Autodesk Fusion 360 part; units mm, degrees
(part 2 of 2)
  spline S93 degree 3 poles (-0.4829, 17.1605) (-0.5355, 17.2267) (-0.6438, 17.3632) (-0.6565, 17.5373) (-0.663, 17.6271) knots 0 0 0 0 0.024747 0.051056 0.051056 0.051056 0.051056
  spline S94 degree 3 poles (-0.663, 17.6271) (-0.6569, 17.7139) (-0.645, 17.8842) (-0.5509, 18.0265) (-0.5048, 18.0964) knots 0 0 0 0 0.025614 0.050281 0.050281 0.050281 0.050281
  spline S95 degree 3 poles (-0.5048, 18.0964) (-0.4337, 18.1672) (-0.2885, 18.3119) (-0.0839, 18.33) (0.0205, 18.3392) knots 0 0 0 0 0.029141 0.059529 0.059529 0.059529 0.059529
  line L42 (4.4066, 19.7731) -> (4.2483, 19.7731)
  line L43 (4.2483, 19.7731) -> (4.2483, 21.7813)
  line L44 (4.2483, 21.7813) -> (4.4939, 21.7813)
  line L45 (4.4939, 21.7813) -> (4.4939, 20.2164)
  spline S96 degree 3 poles (4.4939, 20.2164) (4.5274, 20.2456) (4.5999, 20.3087) (4.6822, 20.3587) (4.7265, 20.3856) knots 0 0 0 0 0.013289 0.028808 0.028808 0.028808 0.028808
  spline S97 degree 3 poles (4.7265, 20.3856) (4.7715, 20.4114) (4.855, 20.4592) (4.944, 20.4957) (4.985, 20.5125) knots 0 0 0 0 0.015536 0.028826 0.028826 0.028826 0.028826
  line L46 (4.985, 20.5125) -> (4.985, 20.2751)
  spline S98 degree 3 poles (4.985, 20.2751) (4.9192, 20.2417) (4.7906, 20.1765) (4.6792, 20.0851) (4.6249, 20.0405) knots 0 0 0 0 0.022076 0.0431 0.0431 0.0431 0.0431
  spline S99 degree 3 poles (4.6249, 20.0405) (4.5785, 19.9972) (4.4934, 19.918) (4.4337, 19.8184) (4.4066, 19.7731) knots 0 0 0 0 0.01891 0.03467 0.03467 0.03467 0.03467
  spline S100 degree 3 poles (-4.5976, 21.8167) (-4.5145, 21.8111) (-4.3537, 21.8001) (-4.2234, 21.7056) (-4.1603, 21.6598) knots 0 0 0 0 0.024413 0.047298 0.047298 0.047298 0.047298
  spline S101 degree 3 poles (-4.1603, 21.6598) (-4.1085, 21.6029) (-4.0028, 21.4869) (-3.9757, 21.3321) (-3.9618, 21.2533) knots 0 0 0 0 0.022603 0.04608 0.04608 0.04608 0.04608
  line L47 (-3.9618, 21.2533) -> (-4.2074, 21.2205)
  spline S102 degree 3 poles (-4.2074, 21.2205) (-4.2215, 21.2828) (-4.2469, 21.3945) (-4.3193, 21.4825) (-4.3513, 21.5214) knots 0 0 0 0 0.018844 0.033755 0.033755 0.033755 0.033755
  spline S103 degree 3 poles (-4.3513, 21.5214) (-4.3875, 21.5482) (-4.461, 21.6029) (-4.5524, 21.6099) (-4.5989, 21.6134) knots 0 0 0 0 0.01322 0.026904 0.026904 0.026904 0.026904
  spline S104 degree 3 poles (-4.5989, 21.6134) (-4.6543, 21.6086) (-4.7643, 21.5989) (-4.8493, 21.5284) (-4.8916, 21.4934) knots 0 0 0 0 0.016258 0.032307 0.032307 0.032307 0.032307
  spline S105 degree 3 poles (-4.8916, 21.4934) (-4.9264, 21.4506) (-4.9969, 21.3639) (-5.0062, 21.2524) (-5.0109, 21.196) knots 0 0 0 0 0.016147 0.032721 0.032721 0.032721 0.032721
  spline S106 degree 3 poles (-5.0109, 21.196) (-5.0068, 21.1425) (-4.9986, 21.038) (-4.9327, 20.9567) (-4.9004, 20.917) knots 0 0 0 0 0.015678 0.030648 0.030648 0.030648 0.030648
  spline S107 degree 3 poles (-4.9004, 20.917) (-4.8604, 20.885) (-4.7783, 20.8193) (-4.6732, 20.8113) (-4.6194, 20.8072) knots 0 0 0 0 0.015012 0.030805 0.030805 0.030805 0.030805
  spline S108 degree 3 poles (-4.6194, 20.8072) (-4.5933, 20.8087) (-4.5347, 20.8122) (-4.4777, 20.8265) (-4.4461, 20.8345) knots 0 0 0 0 0.00784 0.017573 0.017573 0.017573 0.017573
  line L48 (-4.4461, 20.8345) -> (-4.4734, 20.6189)
  spline S109 degree 3 poles (-4.4734, 20.6189) (-4.4808, 20.6197) (-4.494, 20.6211) (-4.5072, 20.6215) (-4.513, 20.6216) knots 0 0 0 0 0.002226 0.003967 0.003967 0.003967 0.003967
  spline S110 degree 3 poles (-4.513, 20.6216) (-4.5637, 20.6184) (-4.6639, 20.612) (-4.7519, 20.5637) (-4.7954, 20.5398) knots 0 0 0 0 0.015044 0.029725 0.029725 0.029725 0.029725
  spline S111 degree 3 poles (-4.7954, 20.5398) (-4.832, 20.5078) (-4.9081, 20.4411) (-4.9165, 20.34) (-4.9209, 20.2874) knots 0 0 0 0 0.014029 0.029194 0.029194 0.029194 0.029194
  spline S112 degree 3 poles (-4.9209, 20.2874) (-4.9173, 20.2446) (-4.9104, 20.1603) (-4.8561, 20.0955) (-4.8295, 20.0637) knots 0 0 0 0 0.012556 0.024703 0.024703 0.024703 0.024703
  spline S113 degree 3 poles (-4.8295, 20.0637) (-4.796, 20.0378) (-4.7266, 19.9842) (-4.6389, 19.9781) (-4.5935, 19.975) knots 0 0 0 0 0.012404 0.025721 0.025721 0.025721 0.025721
  spline S114 degree 3 poles (-4.5935, 19.975) (-4.5481, 19.9783) (-4.4596, 19.9849) (-4.3891, 20.0388) (-4.3547, 20.065) knots 0 0 0 0 0.013323 0.026012 0.026012 0.026012 0.026012
  spline S115 degree 3 poles (-4.3547, 20.065) (-4.3254, 20.1011) (-4.2612, 20.1801) (-4.2423, 20.2805) (-4.2319, 20.3351) knots 0 0 0 0 0.013719 0.030088 0.030088 0.030088 0.030088
  line L49 (-4.2319, 20.3351) -> (-3.9864, 20.2915)
  spline S116 degree 3 poles (-3.9864, 20.2915) (-4.0047, 20.2151) (-4.0397, 20.0694) (-4.1423, 19.9605) (-4.191, 19.9088) knots 0 0 0 0 0.023119 0.04407 0.04407 0.04407 0.04407
  spline S117 degree 3 poles (-4.191, 19.9088) (-4.2487, 19.8692) (-4.3683, 19.7873) (-4.5131, 19.7779) (-4.588, 19.7731) knots 0 0 0 0 0.020598 0.042654 0.042654 0.042654 0.042654
  spline S118 degree 3 poles (-4.588, 19.7731) (-4.6412, 19.7758) (-4.7459, 19.7812) (-4.8421, 19.8228) (-4.8895, 19.8433) knots 0 0 0 0 0.015821 0.03118 0.03118 0.03118 0.03118
  spline S119 degree 3 poles (-4.8895, 19.8433) (-4.9324, 19.8684) (-5.0164, 19.9174) (-5.0728, 19.9964) (-5.1003, 20.035) knots 0 0 0 0 0.014725 0.02878 0.02878 0.02878 0.02878
  spline S120 degree 3 poles (-5.1003, 20.035) (-5.1216, 20.0759) (-5.1637, 20.1568) (-5.1701, 20.2478) (-5.1733, 20.2928) knots 0 0 0 0 0.013662 0.027054 0.027054 0.027054 0.027054
  spline S121 degree 3 poles (-5.1733, 20.2928) (-5.1704, 20.335) (-5.1648, 20.4188) (-5.124, 20.4923) (-5.1037, 20.5289) knots 0 0 0 0 0.012502 0.024877 0.024877 0.024877 0.024877
  spline S122 degree 3 poles (-5.1037, 20.5289) (-5.0768, 20.5629) (-5.0205, 20.6342) (-4.9398, 20.6761) (-4.8977, 20.698) knots 0 0 0 0 0.012871 0.026927 0.026927 0.026927 0.026927
  spline S123 degree 3 poles (-4.8977, 20.698) (-4.953, 20.7146) (-5.0601, 20.7468) (-5.1364, 20.8284) (-5.1733, 20.8679) knots 0 0 0 0 0.016967 0.032892 0.032892 0.032892 0.032892
  spline S124 degree 3 poles (-5.1733, 20.8679) (-5.2019, 20.915) (-5.2621, 21.0139) (-5.2683, 21.1298) (-5.2715, 21.1905) knots 0 0 0 0 0.016275 0.034197 0.034197 0.034197 0.034197
  spline S125 degree 3 poles (-5.2715, 21.1905) (-5.2635, 21.2746) (-5.2474, 21.443) (-5.1362, 21.5707) (-5.0805, 21.6346) knots 0 0 0 0 0.024665 0.049435 0.049435 0.049435 0.049435
  spline S126 degree 3 poles (-5.0805, 21.6346) (-5.0113, 21.6877) (-4.869, 21.797) (-4.6897, 21.81) (-4.5976, 21.8167) knots 0 0 0 0 0.025577 0.052634 0.052634 0.052634 0.052634
  spline S127 degree 3 poles (0, 25.2779) (0.0905, 25.2701) (0.267, 25.2551) (0.3929, 25.131) (0.4543, 25.0705) knots 0 0 0 0 0.026334 0.051363 0.051363 0.051363 0.051363
  spline S128 degree 3 poles (0.4543, 25.0705) (0.5117, 24.9633) (0.6467, 24.7108) (0.6501, 24.423) (0.6521, 24.2574) knots 0 0 0 0 0.036009 0.08476 0.08476 0.08476 0.08476
  spline S129 degree 3 poles (0.6521, 24.2574) (0.6507, 24.1501) (0.6481, 23.9568) (0.6003, 23.7697) (0.5791, 23.6865) knots 0 0 0 0 0.032061 0.057736 0.057736 0.057736 0.057736
  spline S130 degree 3 poles (0.5791, 23.6865) (0.5533, 23.6197) (0.5043, 23.4931) (0.4078, 23.3979) (0.3622, 23.3529) knots 0 0 0 0 0.021191 0.040192 0.040192 0.040192 0.040192
  spline S131 degree 3 poles (0.3622, 23.3529) (0.3097, 23.3187) (0.1997, 23.2471) (0.0685, 23.2395) (0, 23.2356) knots 0 0 0 0 0.018481 0.038665 0.038665 0.038665 0.038665
  spline S132 degree 3 poles (0, 23.2356) (-0.0511, 23.2378) (-0.1493, 23.2421) (-0.2393, 23.2815) (-0.2824, 23.3004) knots 0 0 0 0 0.015196 0.029197 0.029197 0.029197 0.029197
  spline S133 degree 3 poles (-0.2824, 23.3004) (-0.3213, 23.3246) (-0.4002, 23.3739) (-0.4551, 23.4491) (-0.4829, 23.4873) knots 0 0 0 0 0.013619 0.027641 0.027641 0.027641 0.027641
  spline S134 degree 3 poles (-0.4829, 23.4873) (-0.5083, 23.5316) (-0.5619, 23.6256) (-0.5915, 23.7297) (-0.6071, 23.7847) knots 0 0 0 0 0.01527 0.032333 0.032333 0.032333 0.032333
  spline S135 degree 3 poles (-0.6071, 23.7847) (-0.6202, 23.8531) (-0.65, 24.0091) (-0.6514, 24.1681) (-0.6521, 24.2574) knots 0 0 0 0 0.020858 0.04757 0.04757 0.04757 0.04757
  spline S136 degree 3 poles (-0.6521, 24.2574) (-0.6507, 24.364) (-0.648, 24.5564) (-0.6008, 24.7426) (-0.5798, 24.8256) knots 0 0 0 0 0.031856 0.057454 0.057454 0.057454 0.057454
  spline S137 degree 3 poles (-0.5798, 24.8256) (-0.5541, 24.8924) (-0.5054, 25.0192) (-0.4091, 25.1147) (-0.3636, 25.1598) knots 0 0 0 0 0.021185 0.040213 0.040213 0.040213 0.040213
  spline S138 degree 3 poles (-0.3636, 25.1598) (-0.3109, 25.1942) (-0.2006, 25.2663) (-0.0689, 25.2739) (0, 25.2779) knots 0 0 0 0 0.018535 0.038823 0.038823 0.038823 0.038823
  arc A0 (6.725, 12.125) -> (6.925, 12.325) centre (6.725, 12.325) ccw
  line L50 (6.925, 12.325) -> (6.925, 25.775)
  arc A1 (6.925, 25.775) -> (6.725, 25.975) centre (6.725, 25.775) ccw
  line L51 (6.725, 25.975) -> (-6.725, 25.975)
  arc A2 (-6.725, 25.975) -> (-6.925, 25.775) centre (-6.725, 25.775) ccw
  line L52 (-6.925, 25.775) -> (-6.925, 12.325)
  arc A3 (-6.925, 12.325) -> (-6.725, 12.125) centre (-6.725, 12.325) ccw
  line L53 (-6.725, 12.125) -> (6.725, 12.125)
  spline S139 degree 3 poles (0.0027, 23.4388) (0.0564, 23.4451) (0.165, 23.4576) (0.2367, 23.5403) (0.2729, 23.5821) knots 0 0 0 0 0.015627 0.031586 0.031586 0.031586 0.031586
  spline S140 degree 3 poles (0.2729, 23.5821) (0.3095, 23.6678) (0.4012, 23.8822) (0.4003, 24.1166) (0.3997, 24.2574) knots 0 0 0 0 0.027708 0.069337 0.069337 0.069337 0.069337
  spline S141 degree 3 poles (0.3997, 24.2574) (0.4011, 24.3964) (0.4034, 24.6233) (0.3177, 24.832) (0.2844, 24.9129) knots 0 0 0 0 0.041114 0.067132 0.067132 0.067132 0.067132
  spline S142 degree 3 poles (0.2844, 24.9129) (0.2453, 24.9604) (0.1706, 25.051) (0.055, 25.0679) (0, 25.0759) knots 0 0 0 0 0.017756 0.03385 0.03385 0.03385 0.03385
  spline S143 degree 3 poles (0, 25.0759) (-0.055, 25.0679) (-0.1708, 25.0508) (-0.2453, 24.9599) (-0.2844, 24.9122) knots 0 0 0 0 0.016099 0.03389 0.03389 0.03389 0.03389
  spline S144 degree 3 poles (-0.2844, 24.9122) (-0.3177, 24.8313) (-0.4033, 24.6228) (-0.4011, 24.3961) (-0.3997, 24.2574) knots 0 0 0 0 0.026034 0.067063 0.067063 0.067063 0.067063
  spline S145 degree 3 poles (-0.3997, 24.2574) (-0.4012, 24.1181) (-0.4035, 23.8909) (-0.3177, 23.682) (-0.2844, 23.6012) knots 0 0 0 0 0.041199 0.067201 0.067201 0.067201 0.067201
  spline S146 degree 3 poles (-0.2844, 23.6012) (-0.245, 23.5539) (-0.1694, 23.4632) (-0.053, 23.4467) (0.0027, 23.4388) knots 0 0 0 0 0.01777 0.034058 0.034058 0.034058 0.034058
  line L54 (4.4407, 16.713) -> (5.0669, 17.6148)
  line L55 (5.0669, 17.6148) -> (4.4407, 17.6148)
  line L56 (4.4407, 17.6148) -> (4.4407, 16.713)
  spline S147 degree 3 poles (-4.6371, 17.2383) (-4.5838, 17.2432) (-4.477, 17.2532) (-4.3955, 17.3228) (-4.3547, 17.3576) knots 0 0 0 0 0.015669 0.031337 0.031337 0.031337 0.031337
  spline S148 degree 3 poles (-4.3547, 17.3576) (-4.3209, 17.4018) (-4.2503, 17.494) (-4.2427, 17.6102) (-4.2388, 17.6707) knots 0 0 0 0 0.016309 0.034061 0.034061 0.034061 0.034061
  spline S149 degree 3 poles (-4.2388, 17.6707) (-4.241, 17.7126) (-4.2456, 17.7965) (-4.2769, 17.8745) (-4.2927, 17.9136) knots 0 0 0 0 0.012488 0.025026 0.025026 0.025026 0.025026
  spline S150 degree 3 poles (-4.2927, 17.9136) (-4.3119, 17.9496) (-4.3493, 18.0196) (-4.4127, 18.0672) (-4.4434, 18.0902) knots 0 0 0 0 0.012088 0.023476 0.023476 0.023476 0.023476
  spline S151 degree 3 poles (-4.4434, 18.0902) (-4.4757, 18.1079) (-4.5392, 18.1427) (-4.6113, 18.1482) (-4.6467, 18.1509) knots 0 0 0 0 0.01092 0.021432 0.021432 0.021432 0.021432
  spline S152 degree 3 poles (-4.6467, 18.1509) (-4.6971, 18.1453) (-4.8002, 18.1336) (-4.8756, 18.062) (-4.9141, 18.0254) knots 0 0 0 0 0.014798 0.030269 0.030269 0.030269 0.030269
  spline S153 degree 3 poles (-4.9141, 18.0254) (-4.9467, 17.9777) (-5.0166, 17.8752) (-5.0227, 17.7508) (-5.0259, 17.6844) knots 0 0 0 0 0.017015 0.03652 0.03652 0.03652 0.03652
  spline S154 degree 3 poles (-5.0259, 17.6844) (-5.0227, 17.6205) (-5.0166, 17.5007) (-4.9476, 17.4031) (-4.9154, 17.3576) knots 0 0 0 0 0.018742 0.035129 0.035129 0.035129 0.035129
  spline S155 degree 3 poles (-4.9154, 17.3576) (-4.876, 17.3228) (-4.7963, 17.2526) (-4.6905, 17.2431) (-4.6371, 17.2383) knots 0 0 0 0 0.015362 0.030997 0.030997 0.030997 0.030997
  spline S156 degree 3 poles (-4.6112, 13.9613) (-4.6653, 13.9566) (-4.7718, 13.9474) (-4.852, 13.8767) (-4.8916, 13.8419) knots 0 0 0 0 0.01582 0.031195 0.031195 0.031195 0.031195
  spline S157 degree 3 poles (-4.8916, 13.8419) (-4.9236, 13.796) (-4.9926, 13.697) (-4.9983, 13.576) (-5.0014, 13.5111) knots 0 0 0 0 0.01645 0.035493 0.035493 0.035493 0.035493
  spline S158 degree 3 poles (-5.0014, 13.5111) (-4.998, 13.4458) (-4.9917, 13.323) (-4.9216, 13.2225) (-4.8888, 13.1755) knots 0 0 0 0 0.019171 0.036033 0.036033 0.036033 0.036033
  spline S159 degree 3 poles (-4.8888, 13.1755) (-4.8499, 13.1393) (-4.7732, 13.068) (-4.6692, 13.0568) (-4.618, 13.0513) knots 0 0 0 0 0.015505 0.030512 0.030512 0.030512 0.030512
  spline S160 degree 3 poles (-4.618, 13.0513) (-4.5647, 13.0575) (-4.4549, 13.0702) (-4.3743, 13.1461) (-4.3329, 13.185) knots 0 0 0 0 0.015674 0.03225 0.03225 0.03225 0.03225
  spline S161 degree 3 poles (-4.3329, 13.185) (-4.2975, 13.2344) (-4.2234, 13.3378) (-4.2156, 13.465) (-4.2115, 13.5316) knots 0 0 0 0 0.017846 0.037388 0.037388 0.037388 0.037388
  spline S162 degree 3 poles (-4.2115, 13.5316) (-4.2155, 13.5914) (-4.2232, 13.7065) (-4.2932, 13.798) (-4.3268, 13.8419) knots 0 0 0 0 0.017547 0.033771 0.033771 0.033771 0.033771
  spline S163 degree 3 poles (-4.3268, 13.8419) (-4.3676, 13.8767) (-4.4497, 13.9468) (-4.5572, 13.9564) (-4.6112, 13.9613) knots 0 0 0 0 0.015682 0.031535 0.031535 0.031535 0.031535
  spline S164 degree 3 poles (0.0055, 13.8781) (0.0603, 13.8825) (0.168, 13.8911) (0.2516, 13.9593) (0.2926, 13.9927) knots 0 0 0 0 0.016099 0.03158 0.03158 0.03158 0.03158
  spline S165 degree 3 poles (0.2926, 13.9927) (0.3259, 14.0337) (0.3935, 14.1173) (0.4021, 14.2246) (0.4065, 14.2792) knots 0 0 0 0 0.015466 0.031479 0.031479 0.031479 0.031479
  spline S166 degree 3 poles (0.4065, 14.2792) (0.4044, 14.3141) (0.4, 14.3848) (0.3713, 14.4496) (0.3568, 14.4824) knots 0 0 0 0 0.010409 0.021077 0.021077 0.021077 0.021077
  spline S167 degree 3 poles (0.3568, 14.4824) (0.3381, 14.5134) (0.3005, 14.5755) (0.2394, 14.6148) (0.2087, 14.6346) knots 0 0 0 0 0.010689 0.021477 0.021477 0.021477 0.021477
  spline S168 degree 3 poles (0.2087, 14.6346) (0.1753, 14.6503) (0.1083, 14.6818) (0.0343, 14.6862) (-0.0027, 14.6884) knots 0 0 0 0 0.01097 0.022 0.022 0.022 0.022
  spline S169 degree 3 poles (-0.0027, 14.6884) (-0.0583, 14.6842) (-0.1669, 14.676) (-0.2519, 14.6082) (-0.2933, 14.5752) knots 0 0 0 0 0.016312 0.031835 0.031835 0.031835 0.031835
  spline S170 degree 3 poles (-0.2933, 14.5752) (-0.3267, 14.5343) (-0.3951, 14.4505) (-0.4036, 14.3426) (-0.4079, 14.2874) knots 0 0 0 0 0.015466 0.031649 0.031649 0.031649 0.031649
  spline S171 degree 3 poles (-0.4079, 14.2874) (-0.4034, 14.2312) (-0.3945, 14.121) (-0.3243, 14.0358) (-0.2899, 13.994) knots 0 0 0 0 0.016467 0.032302 0.032302 0.032302 0.032302
  spline S172 degree 3 poles (-0.2899, 13.994) (-0.2475, 13.9602) (-0.1611, 13.8912) (-0.0508, 13.8825) (0.0055, 13.8781) knots 0 0 0 0 0.015878 0.032386 0.032386 0.032386 0.032386
  spline S173 degree 3 poles (0.0014, 13.05) (0.0458, 13.0534) (0.1328, 13.06) (0.2012, 13.1138) (0.2347, 13.14) knots 0 0 0 0 0.013054 0.025513 0.025513 0.025513 0.025513
  spline S174 degree 3 poles (0.2347, 13.14) (0.2617, 13.1713) (0.3154, 13.2334) (0.3234, 13.3151) (0.3274, 13.3556) knots 0 0 0 0 0.012093 0.023986 0.023986 0.023986 0.023986
  spline S175 degree 3 poles (0.3274, 13.3556) (0.3241, 13.4002) (0.3175, 13.4872) (0.2627, 13.5547) (0.236, 13.5875) knots 0 0 0 0 0.013093 0.025466 0.025466 0.025466 0.025466
  spline S176 degree 3 poles (0.236, 13.5875) (0.2025, 13.6137) (0.1328, 13.6682) (0.0444, 13.6744) (-0.0014, 13.6775) knots 0 0 0 0 0.012488 0.025912 0.025912 0.025912 0.025912
  spline S177 degree 3 poles (-0.0014, 13.6775) (-0.046, 13.6743) (-0.1328, 13.668) (-0.2009, 13.6142) (-0.234, 13.5882) knots 0 0 0 0 0.013101 0.025433 0.025433 0.025433 0.025433
  spline S178 degree 3 poles (-0.234, 13.5882) (-0.2604, 13.5566) (-0.3136, 13.4932) (-0.321, 13.4107) (-0.3247, 13.3692) knots 0 0 0 0 0.012047 0.024215 0.024215 0.024215 0.024215
  spline S179 degree 3 poles (-0.3247, 13.3692) (-0.3209, 13.3261) (-0.3135, 13.2406) (-0.2585, 13.1747) (-0.2312, 13.1421) knots 0 0 0 0 0.012649 0.025094 0.025094 0.025094 0.025094
  spline S180 degree 3 poles (-0.2312, 13.1421) (-0.1978, 13.1152) (-0.1298, 13.0606) (-0.0428, 13.0536) (0.0014, 13.05) knots 0 0 0 0 0.012558 0.025536 0.025536 0.025536 0.025536
component "Plate" placed x (1, 0, 0) y (0, 1, 0) z (0, 0, 1) at (0, 0, 0)
component "Insert" placed x (1, 0, 0) y (0, 1, 0) z (0, 0, 1) at (0, 0, 0) in component "Plate"
equation "WallThickness = 5 mm"
equation "d24 = 80 mm + ( WallThickness * 2 ) + 5 mm"
equation "d25 = WallThickness * 2"
equation "d35 = WallThickness * 2"
